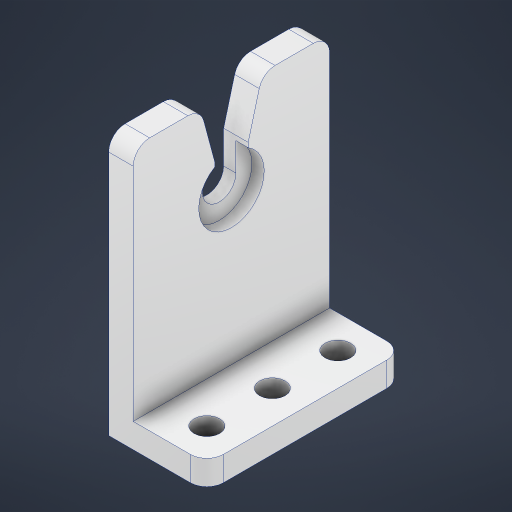
# Autodesk Inventor part: BUMP_007_Smallbracket
Saved by Autodesk Inventor 2024.2 (Build 282272000, 272)
## iProperties
Created: 2024-08-10
Part Number: BUMP_007_Smallbracket
Material: Aluminum 6061
Document SubType Name: Modeling
Designer: Bryan
Density: 2.7 g/cm^3
Appearance: Aluminum - Flat
Mass: 28.818 g
Surface Area: 58.3399 cm^2
Volume: 10.6733 cm^3
Author: Bryan
Autodesk Inventor part; units mm, degrees
ref_plane "YZ Plane" through (0, 0, 0) normal (1, 0, 0) x (0, 1, 0)
ref_plane "XZ Plane" through (0, 0, 0) normal (0, 1, 0) x (-1, 0, 0)
ref_plane "XY Plane" through (0, 0, 0) normal (0, 0, 1) x (1, 0, 0)
sketch "Sketch2" plane through (0, 0, 0) normal (0, 0, 1) x (1, 0, 0)
  line L0 (0, 0) -> (0, 50.8)
  line L1 (0, 50.8) -> (4.7625, 50.8)
  line L2 (4.7625, 50.8) -> (4.7625, 4.7625)
  line L3 (4.7625, 4.7625) -> (19.05, 4.7625)
  line L4 (19.05, 4.7625) -> (19.05, 0)
  line L5 (19.05, 0) -> (0, 0)
  dimension "d0" = 4.7625
  dimension "d1" = 50.8
  dimension "d2" = 19.05
  constraints: 12 end point, 3 horizontal, 3 vertical, 1 perpendicular
  measures "d0" distance of L0.end L1.end
  measures "d1" distance of L0.start L0.end
  measures "d2" distance of L4.end L0.start
extrude "Extrusion1" add sketch "Sketch2" along normal blind 38.1
sketch "Sketch3" plane through (4.7625, 4.7625, 0) normal (1, 0, 0) x (0, 0, -1)
  circle A0 centre (-19.05, 29.3688) radius 3.2512
  line L0 (-22.3012, 29.3688) -> (-22.3012, 35.7188)
  line L1 (-22.3012, 35.7188) -> (-25.0661, 46.0375)
  line L2 (0, 46.0375) -> (-38.1, 46.0375) projected
  line L3 (-13.0339, 46.0375) -> (-15.7988, 35.7188)
  line L4 (-15.7988, 35.7188) -> (-15.7988, 29.3688)
  line L5 (-38.1, 0) -> (-38.1, 46.0375) projected
  point P0 (0, -4.7625)
  point P1 (-19.05, 46.0375)
  point P2 (-38.1, 23.0187)
  point P3 (-38.1, 23.0187)
  dimension "d5" = 6.5024
  dimension "d6" = 165
  dimension "d7" = 6.35
  dimension "d18" = 6.35
  constraints: 8 end point, 3 midpoint, 2 equal length, 2 point on circle, 2 point on line, 2 tangent, 1 centre point, 1 parallel, 1 vertical, 1 vertical alignment
  measures "d5" diameter of A0
  measures "d6" angle of L0 L1
  measures "d7" distance of L0.start L0.end
  measures "d18" vertical distance of point (-38.1, 23.019) A0.centre
extrude "Extrusion2" cut sketch "Sketch3" against normal blind 38.1
sketch "Sketch4" plane through (4.7625, 4.7625, 0) normal (0, 1, 0) x (1, 0, 0)
  circle A0 centre (7.9375, -31.75) radius 2.4892
  circle A1 centre (7.9375, -6.35) radius 2.4892
  line L0 (14.2875, -38.1) -> (0, -38.1) projected
  line L1 (14.2875, 0) -> (0, 0) projected
  circle A2 centre (7.9375, -19.05) radius 2.4892
  line L2 (-4.7625, -25.0661) -> (-4.7625, -38.1) projected
  point P0 (-4.7625, 0)
  point P1 (7.1437, -38.1)
  dimension "d10" = 4.9784
  dimension "d11" = 4.9784
  dimension "d12" = 6.35
  dimension "d13" = 6.35
  dimension "d14" = 25.4
  dimension "d22" = 12.7
  dimension "d23" = 12.7
  constraints: 3 centre point, 2 vertical alignment, 1 equal radius, 1 midpoint
  measures "d10" diameter of A0
  measures "d11" diameter of A1
  measures "d12" vertical distance of point (7.144, -38.1) A0.centre
  measures "d13" distance from line of L1 A1.centre
  measures "d14" distance of A1.centre A0.centre
  measures "d22" distance from line of L2 A0.centre
  measures "d23" distance of A1.centre A2.centre
extrude "Extrusion3" cut sketch "Sketch4" against normal blind 38.1
fillet "Fillet1" radius 3.175 6 edges at (2.3813, 50.8, 38.1) (2.3813, 50.8, 25.0661) (2.3813, 50.8, 13.0339) (2.3813, 50.8, 0) (19.05, 2.3813, 38.1) (19.05, 2.3813, 0)
sketch "Sketch5" plane through (4.7625, 4.7625, 38.1) normal (1, 0, 0) x (0, 0, -1)
  arc A0 (15.7988, 29.3688) -> (22.3012, 29.3688) centre (19.05, 29.3688) ccw projected
  circle A1 centre (19.05, 29.3688) radius 6.35
  point P0 (38.1, -4.7625)
  dimension "d19" = 12.7
  constraints: 1 centre point, 1 coincident
  measures "d19" diameter of A1
extrude "Extrusion4" cut sketch "Sketch5" against normal blind 2.3813
equation "\"d13\" = d12"
body "Solid1"
